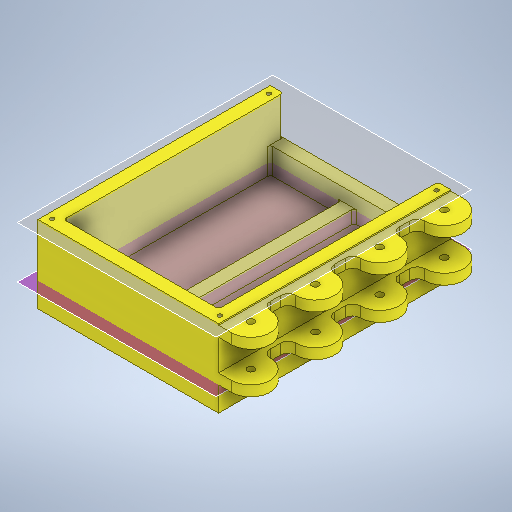
# Autodesk Inventor part: акб корпус
Saved by Autodesk Inventor 2025 (Build 290162000, 162)
## iProperties
Created: 2025-02-25
Part Number: акб корпус
Material: Пластик АБС
Document SubType Name: Modeling
Designer: volko
Density: 1.06 g/cm^3
Appearance: Канареечный
Mass: 569.222 g
Surface Area: 1154.58 cm^2
Volume: 537.002 cm^3
Author: volko
Autodesk Inventor part; units mm, degrees
ref_plane "YZ Plane" through (0, 0, 0) normal (1, 0, 0) x (0, 1, 0)
ref_plane "XZ Plane" through (0, 0, 0) normal (0, 1, 0) x (-1, 0, 0)
ref_plane "XY Plane" through (0, 0, 0) normal (0, 0, 1) x (1, 0, 0)
sketch "Эскиз1" plane through (0, 0, 0) normal (0, 1, 0) x (-1, 0, 0)
  line L0 (60, 80) -> (-60, 80)
  line L1 (-60, 80) -> (-60, -80)
  line L2 (-60, -80) -> (60, -80)
  line L3 (60, -80) -> (60, 80)
  line L4 (-70, 94) -> (-70, -94) construction
  line L5 (-70, -90) -> (70, -90)
  line L6 (70, -94) -> (70, 94) construction
  line L7 (-99.2334, 0) -> (99.2334, 0) projected
  line L8 (0, -144.1107) -> (0, 144.1107) projected
  line L9 (5, -80) -> (-5, -80)
  line L10 (-5, -80) -> (-5, 80)
  line L11 (-5, 80) -> (5, 80)
  line L12 (5, 80) -> (5, -80)
  arc A0 (-54.254, 96) -> (-70, 94) centre (-62, 94) ccw construction
  arc A1 (-54.254, 96) -> (-46.5081, 90) centre (-46.5081, 98) ccw construction
  line L13 (70, 90) -> (-70, 90)
  arc A2 (70, 94) -> (54.254, 96) centre (62, 94) ccw construction
  arc A3 (46.5081, 90) -> (54.254, 96) centre (46.5081, 98) ccw construction
  arc A4 (-70, -94) -> (-54.254, -96) centre (-62, -94) ccw construction
  arc A5 (-46.5081, -90) -> (-54.254, -96) centre (-46.5081, -98) ccw construction
  arc A6 (54.254, -96) -> (46.5081, -90) centre (46.5081, -98) ccw construction
  arc A7 (54.254, -96) -> (70, -94) centre (62, -94) ccw construction
  line L14 (70, -90) -> (70, 90)
  line L15 (-70, -90) -> (-70, 90)
  point P0 (0, 0)
  point P1 (5, 80)
  point P2 (-5, -80)
  dimension "d12" = 160
  dimension "d14" = 55
  dimension "d15" = 10
  dimension "d16" = 10
  dimension "d17" = 10
  dimension "d70" = 8
  dimension "d71" = 4
  constraints: 28 end point, 16 point on circle, 15 symmetric about line, 10 point on line, 8 centre point, 6 parallel, 4 perpendicular, 3 horizontal, 3 tangent, 1 collinear, 1 equal radius, 11 other
  measures "d12" distance of L2.end L0.start
  measures "d14" distance between parallel lines of L12 L3
  measures "d15" distance between parallel lines of L10 L12
  measures "d16" distance between parallel lines of L4 L1
  measures "d17" distance between parallel lines of L2 L5
  measures "d70" radius of A0
  measures "d71" distance from line of L13 A0.centre
extrude "Выдавливание2" add sketch "Эскиз1" along normal blind 10
extrude "Выдавливание5" add sketch "Эскиз1" along normal blind 20 contours L12 L7 L8 L0 | L8 L7 L10 L0 | L12 L2 L8 L7 | L8 L2 L10 L7
extrude "Выдавливание7" add sketch "Эскиз1" along normal blind 60 contours L0 L8 L13 L14 L7 L3 | L7 L14 L5 L8 L2 L3 | L0 L1 L7 L15 L13 L8 | L8 L5 L15 L7 L1 L2
ref_plane "РабПлоскость1" through (0, 19, 0) normal (0, -1, 0) x (1, 0, 0)
sketch "Эскиз6" plane through (0, 0, 0) normal (0, 0, 1) x (1, 0, 0)
  line L0 (60, 10) -> (60, 60) projected
  line L1 (-60, 10) -> (-60, 60) projected
  line L2 (60, 60) -> (-60, 60)
  line L3 (-60, 60) -> (-60, 30)
  line L4 (-60, 30) -> (60, 30)
  line L5 (60, 30) -> (60, 60)
  point P0 (0, 0)
  dimension "d30" = 30
  constraints: 8 end point, 2 parallel, 1 horizontal, 1 perpendicular, 1 point on line
  measures "d30" distance between parallel lines of L4 L2
extrude "Выдавливание8" cut sketch "Эскиз6" against normal through all
fillet "Сопряжение3" radius 2 10 edges at (60, 35, 80) (-60, 35, 80) (5, 15, 80) (-5, 15, 80) (5, 15, -80) (60, 20, -80) (-5, 15, -80) (-60, 20, -80) (60, 45, -90) (-60, 45, -90)
sketch "Эскиз9" plane through (0, 19, 0) normal (0, -1, 0) x (1, 0, 0)
  line L0 (24.9995, 90) -> (27, 90)
  line L1 (70, -90) -> (62, -90) projected
  line L2 (70, -90) -> (80, -90)
  line L3 (-102.6, 0) -> (125.6, 0) projected
  arc A0 (80, -90) -> (80, -60) centre (80, -75) ccw
  line L4 (80, -60) -> (80, -60)
  line L5 (74, -54) -> (74, -46)
  arc A1 (80, -40) -> (80, -10) centre (80, -25) ccw
  line L6 (80, -10) -> (80, -10)
  arc A2 (74, -54) -> (80, -60) centre (80, -54) ccw
  line L7 (70, 90) -> (70, -90) projected
  line L8 (80, -40) -> (80, -40)
  arc A3 (80, -40) -> (74, -46) centre (80, -46) ccw
  arc A4 (74, -4) -> (80, -10) centre (80, -4) ccw
  line L9 (74, -4) -> (74, 4)
  line L10 (70, 90) -> (80, 90)
  arc A5 (80, 60) -> (80, 90) centre (80, 75) ccw
  line L11 (74, 54) -> (74, 46)
  arc A6 (80, 10) -> (80, 40) centre (80, 25) ccw
  line L12 (80, 10) -> (80, 10)
  arc A7 (80, 60) -> (74, 54) centre (80, 54) ccw
  arc A8 (74, 46) -> (80, 40) centre (80, 46) ccw
  arc A9 (80, 10) -> (74, 4) centre (80, 4) ccw
  line L13 (80, 40) -> (80, 40)
  line L14 (80, 60) -> (80, 60)
  point P0 (0, 0)
  point P1 (-65, 90)
  point P2 (65, 90)
  point P3 (15, 90)
  point P4 (74, 0)
  dimension "d90" = 15
  dimension "d91" = 6
  dimension "d93" = 10
  constraints: 24 end point, 21 point on circle, 14 symmetric about line, 11 tangent, 10 centre point, 6 horizontal, 4 coincident, 3 equal radius, 2 equal length, 2 point on line, 1 collinear, 1 midpoint, 1 perpendicular, 1 vertical, 5 other
  measures "d90" radius of A0
  measures "d91" radius of A2
  measures "d93" distance from line of L7 A0.centre
sketch "Эскиз8" plane through (0, 60, 0) normal (0, 1, 0) x (1, 0, 0)
  line L0 (0, 140.0952) -> (0, -128.3492) projected
  line L1 (-98, 0) -> (98, 0) projected
  line L2 (-60, -78) -> (-60, 88) projected
  line L3 (-70, -90) -> (70, -90) projected
  point P0 (0, 0)
  point P1 (-65, -84)
  point P2 (-65, 84)
  point P3 (65, -84)
  point P4 (65, 84)
  point P5 (-65, -90)
  point P6 (65, -90)
  point P7 (-60, 101.746)
  point P8 (-46.5081, -90)
  point P9 (46.5081, -90)
  dimension "d60" = 168
  dimension "d63" = 130
  dimension "d66" = 5
  dimension "d67" = 6
  constraints: 1 horizontal, 1 vertical, 3 other
  measures "d60" distance of point (-65, -84) point (-65, 84)
  measures "d63" distance of point (-65, -84) point (65, -84)
  measures "d66" distance from line of point (-65, -84) L2
  measures "d67" distance from line of point (-65, -84) L3
hole "Отверстие2" at (-65, 60, 84) at (65, 60, 84) at (65, 60, -84) at (-65, 60, -84) direction (0, -1, 0) diameter 3.242 depth 11.8 tip angle 118 thread size "M4x0.7" class "6H" standard "ISO Metric profile"
extrude "Выдавливание10" add sketch "Эскиз9" against normal blind 8
ref_plane "РабПлоскость2" through (0, 59, 0) normal (0, 1, 0) x (1, 0, 0)
sketch "Эскиз10" plane through (0, 59, 0) normal (0, 1, 0) x (1, 0, 0)
  arc A0 (80, 60) -> (80, 90) centre (80, 75) ccw projected
  line L0 (80, 90) -> (70, 90) projected
  line L1 (70, -90) -> (70, 90) projected
  line L2 (70, -90) -> (80, -90) projected
  arc A1 (80, -90) -> (80, -60) centre (80, -75) ccw projected
  arc A2 (74, -54) -> (80, -60) centre (80, -54) ccw projected
  line L3 (74, -54) -> (74, -46) projected
  arc A3 (80, -40) -> (74, -46) centre (80, -46) ccw projected
  arc A4 (80, -40) -> (80, -10) centre (80, -25) ccw projected
  arc A5 (74, -4) -> (80, -10) centre (80, -4) ccw projected
  line L4 (74, -4) -> (74, 4) projected
  arc A6 (80, 10) -> (74, 4) centre (80, 4) ccw projected
  arc A7 (80, 10) -> (80, 40) centre (80, 25) ccw projected
  arc A8 (74, 46) -> (80, 40) centre (80, 46) ccw projected
  line L5 (74, 46) -> (74, 54) projected
  arc A9 (80, 60) -> (74, 54) centre (80, 54) ccw projected
  point P0 (0, 0)
extrude "Выдавливание11" add sketch "Эскиз10" against normal blind 8
hole "Отверстие3" at (80, 19, 75) at (80, 19, 25) at (80, 19, -25) at (80, 19, -75) direction (0, 1, 0) diameter 5.5 end through all
